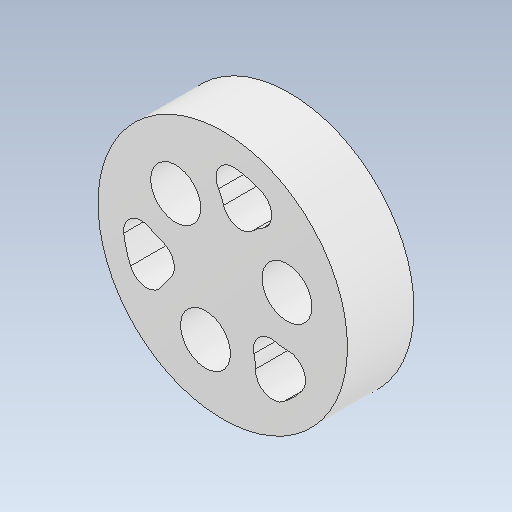
# Autodesk Inventor part: アームカムD15t4
Saved by Autodesk Inventor 2020.2 (Build 242310000, 310)
## iProperties
Created: 2020-03-20
Part Number: アームカムD15t4
Material: アセタール樹脂、白
Document SubType Name: Modeling
Designer: aoyam
Density: 1.425 g/cm^3
Appearance: 滑らか - 白
Mass: 0.8864 g
Surface Area: 6.12611 cm^2
Volume: 0.622035 cm^3
Author: aoyam
Autodesk Inventor part; units mm, degrees
ref_plane "YZ Plane" through (0, 0, 0) normal (1, 0, 0) x (0, 1, 0)
ref_plane "XZ Plane" through (0, 0, 0) normal (0, 1, 0) x (-1, 0, 0)
ref_plane "XY Plane" through (0, 0, 0) normal (0, 0, 1) x (1, 0, 0)
sketch "スケッチ1" plane through (0, 0, 0) normal (0, 0, 1) x (1, 0, 0)
  circle A0 centre (0, 0) radius 6.975
  circle A1 centre (-2.8284, 2.8284) radius 1.5
  circle A2 centre (-1.0353, -3.8637) radius 1.5
  circle A3 centre (3.8637, 1.0353) radius 1.5
  circle A4 centre (0, 0) radius 7.5
  dimension "d0" = 13.95
  dimension "d1" = 3
  dimension "d2" = 4
  dimension "d5" = 360
  dimension "d9" = 15
  constraints: 5 centre point, 2 coincident, 7 other
  measures "d0" diameter of A0
  measures "d1" diameter of A1
  measures "d2" distance of A1.centre point (0, 0)
  measures "d9" diameter of A4
extrude "押し出し2" add sketch "スケッチ1" along normal blind 4 contours A0 | A4
sketch "スケッチ2" plane through (0, 0, 4) normal (0, 0, 1) x (1, 0, 0)
  circle A0 centre (0, 0) radius 7.5 projected
  circle A1 centre (-1.0353, -3.8637) radius 1.5 projected
  circle A2 centre (-2.8284, 2.8284) radius 1.5 projected
  circle A3 centre (3.8637, 1.0353) radius 1.5 projected
  circle A4 centre (0, 0) radius 3
  circle A5 centre (0, 0) radius 6
  circle A6 centre (-2.8284, 2.8284) radius 3
  circle A7 centre (-1.0353, -3.8637) radius 3
  circle A8 centre (3.8637, 1.0353) radius 3
  point P0 (5.882, -1.1843)
  point P1 (2.5106, -1.6422)
  point P2 (1.6422, -2.5106)
  point P3 (1.1843, -5.882)
  point P4 (1.3531, 2.6775)
  point P5 (4.5018, 3.9666)
  point P6 (-1.9153, 5.6861)
  point P7 (0.1669, 2.9954)
  point P8 (-3.9666, -4.5018)
  point P9 (-2.6775, -1.3531)
  point P10 (-2.9954, -0.1669)
  point P11 (-5.6861, 1.9153)
  dimension "d13" = 6
  dimension "d14" = 1.5
  dimension "d15" = 1.5
  dimension "d16" = 1.5
  dimension "d17" = 1.5
  constraints: 5 centre point, 1 coincident
  measures "d13" diameter of A4
  measures "d14" radial gap between concentric circles of A0 A5
  measures "d15" radial gap between concentric circles of A2 A6
  measures "d16" radial gap between concentric circles of A1 A7
  measures "d17" radial gap between concentric circles of A3 A8
extrude "押し出し3" cut sketch "スケッチ2" against normal blind 10 contours A4 A8 A5 A7 | A7 A5 A6 A4 | A4 A6 A5 A8
fillet "フィレット1" radius 1.05 12 edges at (-1.9153, 5.6861, 2) (4.5018, 3.9666, 2) (0.1669, 2.9954, 2) (1.3531, 2.6775, 2) (-5.6861, 1.9153, 2) (-2.9954, -0.1669, 2) (-2.6775, -1.3531, 2) (-3.9666, -4.5018, 2) (2.5106, -1.6422, 2) (1.6422, -2.5106, 2) (5.882, -1.1843, 2) (1.1843, -5.882, 2)
